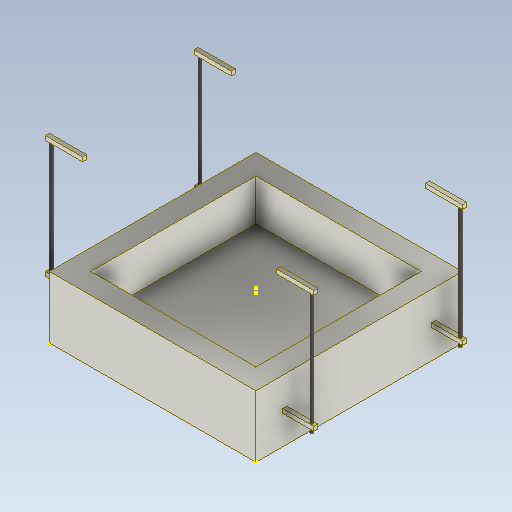
# Autodesk Inventor part: container 1
Saved by Autodesk Inventor 2021 (Build 250183000, 183)
## iProperties
Created: 2021-07-04
Part Number: container 1
Material: Silver
Document SubType Name: Modeling
Designer: Pranali
Density: 10.49 g/cm^3
Appearance: Silver
Author: Pranali
Autodesk Inventor part; units mm, degrees
ref_plane "YZ Plane" through (0, 0, 0) normal (1, 0, 0) x (0, 1, 0)
ref_plane "XZ Plane" through (0, 0, 0) normal (0, 1, 0) x (-1, 0, 0)
ref_plane "XY Plane" through (0, 0, 0) normal (0, 0, 1) x (1, 0, 0)
sketch "Sketch1" plane through (0, 0, 0) normal (0, 1, 0) x (-1, 0, 0)
  line L0 (0, 0) -> (100, 0)
  line L1 (100, 0) -> (100, -100)
  line L2 (100, -100) -> (0, -100)
  line L3 (0, -100) -> (0, 0)
  dimension "d0" = 100
  dimension "d1" = 100
  constraints: 8 end point, 2 parallel, 1 horizontal, 1 perpendicular
  measures "d0" distance of L1.end L2.end
  measures "d1" distance of L0.end L1.end
extrude "Extrusion1" add sketch "Sketch1" along normal blind 30
sketch "Sketch2" plane through (0, 30, 0) normal (0, 1, 0) x (1, 0, 0)
  line L0 (0, 0) -> (0, 100) projected
  line L1 (-100, 0) -> (0, 0) projected
  line L2 (0, 10) -> (0, 0)
  line L3 (-10, 10) -> (-90, 10)
  line L4 (-90, 10) -> (-90, 90)
  line L5 (-90, 90) -> (-10, 90)
  line L6 (-10, 90) -> (-10, 10)
  dimension "d6" = 80
  dimension "d7" = 80
  constraints: 10 end point, 2 parallel, 1 horizontal, 1 perpendicular
  measures "d6" distance of L4.end L5.end
  measures "d7" distance of L3.end L4.end
extrude "Extrusion2" cut sketch "Sketch2" against normal blind 20
sketch "Sketch5" plane through (0, 0, 0) normal (1, 0, 0) x (0, 0, -1)
  point P0 (0, 0)
sketch "Sketch6" plane through (0, 0, 0) normal (1, 0, 0) x (0, 0, -1)
  line L0 (13, 16) -> (15, 16)
  line L1 (15, 16) -> (15, 14)
  line L2 (15, 14) -> (13, 14)
  line L3 (13, 14) -> (13, 16)
  line L4 (13, 16) -> (15, 14) construction
  line L5 (15, 16) -> (13, 14) construction
  line L6 (85, 16) -> (87, 16)
  line L7 (87, 16) -> (87, 14)
  line L8 (87, 14) -> (85, 14)
  line L9 (85, 14) -> (85, 16)
  line L10 (85, 16) -> (87, 14) construction
  line L11 (87, 16) -> (85, 14) construction
  point P0 (0, 0)
  point P1 (14, 15)
  point P2 (86, 15)
  dimension "d22" = 2
  dimension "d23" = 2
  dimension "d24" = 2
  dimension "d25" = 2
  constraints: 24 end point, 4 midpoint, 4 parallel, 2 horizontal, 2 perpendicular
  measures "d22" distance of L1.end L2.end
  measures "d23" distance of L0.end L1.end
  measures "d24" distance of L7.end L8.end
  measures "d25" distance of L6.end L7.end
extrude "Extrusion5" add sketch "Sketch6" along normal blind 15
pattern_linear "Rectangular Pattern1" count 2 spacing 115 along (-1, 0, 0) of "Extrusion5"
sketch "Sketch7" plane through (0, 16, -85) normal (0, 1, 0) x (1, 0, 0)
  circle A0 centre (13, 1) radius 0.75
  point P0 (0, -85)
  dimension "d31" = 1.5
  constraints: 1 centre point
  measures "d31" diameter of A0
extrude "Extrusion6" add sketch "Sketch7" along normal blind 55
sketch "Sketch8" plane through (0, 14, -87) normal (0, -1, 0) x (1, 0, 0)
  circle A0 centre (13, 1) radius 0.75 projected
  circle A1 centre (13, 1) radius 0.75
  point P0 (0, 87)
  dimension "d34" = 1.5
  constraints: 2 coincident, 1 centre point
  measures "d34" diameter of A1
extrude "Extrusion7" add sketch "Sketch8" along normal blind 2
thread "Thread1" size "M1.6x0.35" class "6g" standard "ANSI Metric M Profile" full length
pattern_linear "Rectangular Pattern2" count 2 spacing 72 along (0, 0, 1) of "Extrusion6"
pattern_linear "Rectangular Pattern3" count 2 spacing 126 along (-1, 0, 0) of "Extrusion6", "Rectangular Pattern2"
thread "Thread2" size "M1.6x0.35" class "6g" standard "ANSI Metric M Profile" full length
thread "Thread3" size "M1.6x0.35" class "6g" standard "ANSI Metric M Profile" full length
thread "Thread4" size "M1.6x0.35" class "6g" standard "ANSI Metric M Profile" full length
pattern_linear "Rectangular Pattern4" count 2 spacing 72 along (0, 0, 1) count 2 spacing 126 along (-1, 0, 0) of "Extrusion7"
thread "Thread5" size "M1.6x0.35" class "6g" standard "ANSI Metric M Profile" full length
thread "Thread6" size "M1.6x0.35" class "6g" standard "ANSI Metric M Profile" full length
thread "Thread7" size "M1.6x0.35" class "6g" standard "ANSI Metric M Profile" full length
sketch "Sketch9" plane through (-100, 0, -100) normal (-1, 0, 0) x (0, 0, 1)
  point P0 (100, 0)
sketch "Sketch10" plane through (-113, 71, -14) normal (0, 1, 0) x (1, 0, 0)
  point P0 (113, -14)
sketch "Sketch11" plane through (-113, 71, -86) normal (0, 1, 0) x (1, 0, 0)
  line L0 (-2, -1) -> (-2, 1) projected
  line L1 (-2, 1) -> (16, 1)
  line L2 (16, 1) -> (16, -1)
  line L3 (16, -1) -> (-2, -1)
  line L4 (-2, -1) -> (-2, 1)
  point P0 (113, -86)
  dimension "d63" = 18
  constraints: 8 end point, 2 parallel, 1 horizontal, 1 perpendicular
  measures "d63" distance of L2.end L3.end
extrude "Extrusion8" add sketch "Sketch11" along normal blind 2
sketch "Sketch12" plane through (-113, 73, -86) normal (0, 1, 0) x (1, 0, 0)
  point P0 (113, -86)
sketch "Sketch13" plane through (13, 71, -86) normal (0, 1, 0) x (1, 0, 0)
  line L0 (-13, -1) -> (2, -1) projected
  line L1 (2, -1) -> (-16, -1)
  line L2 (-16, -1) -> (-16, 1)
  line L3 (-16, 1) -> (2, 1)
  line L4 (2, 1) -> (2, -1)
  point P0 (-13, -86)
  dimension "d66" = 18
  dimension "d67" = 2
  constraints: 8 end point, 2 parallel, 1 horizontal, 1 perpendicular
  measures "d66" distance of L2.end L3.end
  measures "d67" distance of L1.end L2.end
extrude "Extrusion9" add sketch "Sketch13" along normal blind 2
pattern_linear "Rectangular Pattern5" count 2 spacing 72 along (0, 0, 1) of "Extrusion9"
pattern_linear "Rectangular Pattern6" count 2 spacing 72 along (0, 0, 1) of "Extrusion8"
body "Solid1"
